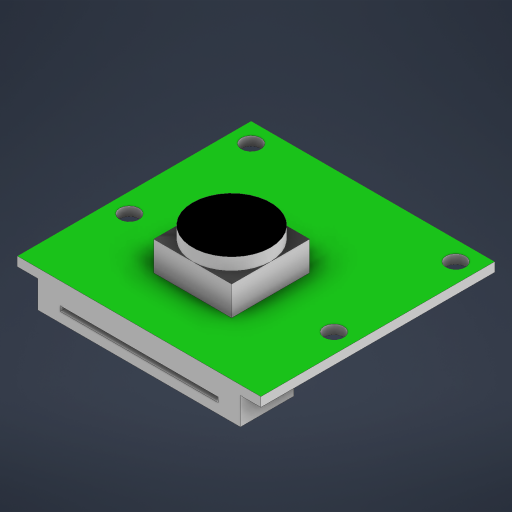
# Autodesk Inventor part: r_camera v2
Saved by Autodesk Inventor 2024.2 (Build 282272000, 272)
## iProperties
Created: 2023-06-18
Part Number: r_camera v2
Material: 일반
Document SubType Name: Modeling
Designer: 6gioc
Density: 1 g/cm^3
Appearance: 기본값
Mass: 1.10891 g
Surface Area: 16.6674 cm^2
Volume: 1.10891 cm^3
Author: 6gioc
Autodesk Inventor part; units mm, degrees
ref_plane "YZ Plane" through (0, 0, 0) normal (1, 0, 0) x (0, 1, 0)
ref_plane "XZ Plane" through (0, 0, 0) normal (0, 1, 0) x (-1, 0, 0)
ref_plane "XY Plane" through (0, 0, 0) normal (0, 0, 1) x (1, 0, 0)
sketch "스케치1" plane through (0, 0, 0) normal (0, 1, 0) x (-1, 0, 0)
  line L0 (0, 0) -> (-25, 0)
  line L1 (-25, 0) -> (-25, -24)
  line L2 (-25, -24) -> (0, -24)
  line L3 (0, -24) -> (0, 0)
  circle A0 centre (-2, -22) radius 1
  circle A1 centre (-23, -22) radius 1
  circle A2 centre (-23, -9.5) radius 1
  circle A3 centre (-2, -9.5) radius 1
  line L4 (-8.5, -13.5) -> (-16.5, -13.5)
  line L5 (-16.5, -13.5) -> (-16.5, -5.5)
  line L6 (-16.5, -5.5) -> (-8.5, -5.5)
  line L7 (-8.5, -5.5) -> (-8.5, -13.5)
  circle A4 centre (-12.5, -9.5) radius 4
  line L8 (-2.1, 0) -> (-22.9, 0)
  line L9 (-22.9, 0) -> (-22.9, -5.5)
  line L10 (-22.9, -5.5) -> (-2.1, -5.5)
  line L11 (-2.1, -5.5) -> (-2.1, 0)
  point P0 (-12.5, 0)
  point P1 (-16.5, -9.5)
  point P2 (-12.5, -5.5)
  point P3 (-8.5, -9.5)
  point P4 (-12.5, -13.5)
  dimension "d0" = 25
  dimension "d1" = 24
  dimension "d2" = 2
  dimension "d3" = 2
  dimension "d4" = 2
  dimension "d5" = 2
  dimension "d6" = 2
  dimension "d8" = 2
  dimension "d9" = 2
  dimension "d10" = 2
  dimension "d12" = 2
  dimension "d15" = 12.5
  dimension "d16" = 9.5
  dimension "d17" = 2
  dimension "d18" = 12.5
  dimension "d19" = 9.5
  dimension "d20" = 8
  dimension "d21" = 8
  dimension "d22" = 8.5
  dimension "d23" = 8.5
  dimension "d24" = 5.5
  dimension "d25" = 21
  dimension "d26" = 8
  dimension "d27" = 20.8
  dimension "d28" = 5.5
  constraints: 24 end point, 6 parallel, 5 centre point, 3 horizontal, 3 perpendicular, 2 midpoint, 2 tangent
  measures "d0" distance of L2.end L1.end
  measures "d1" distance of L1.end L0.end
  measures "d2" diameter of A0
  measures "d3" diameter of A1
  measures "d4" diameter of A2
  measures "d5" diameter of A3
  measures "d6" distance from line of L3 A0.centre
  measures "d8" distance from line of L1 A1.centre
  measures "d9" distance from line of A1.centre L2
  measures "d10" distance from line of L3 A3.centre
  measures "d12" distance from line of L1 A2.centre
  measures "d15" distance of A3.centre A0.centre
  measures "d16" distance from line of L0 A3.centre
  measures "d17" distance from line of L2 A0.centre
  measures "d18" distance of A1.centre A2.centre
  measures "d19" distance from line of L0 A2.centre
  measures "d20" distance of L5.end L6.end
  measures "d21" distance of L4.end L5.end
  measures "d22" distance between parallel lines of L3 L7
  measures "d23" distance between parallel lines of L1 L5
  measures "d24" distance between parallel lines of L0 L6
  measures "d25" distance of A1.centre A0.centre
  measures "d26" diameter of A4
  measures "d27" distance of L10.end L9.end
  measures "d28" distance of L9.end L8.end
extrude "돌출1" add sketch "스케치1" along normal blind 0.95 contours L3 L2 L1 L0 L9 L10 L5 L4 L7 L11 | L11 L10 L6 L9 L0
extrude "돌출2" add sketch "스케치1" along normal blind 3.95 contours L7 A4 L6 | L6 A4 L5 | L7 L4 A4 | A4 L4 L5
extrude "돌출3" add sketch "스케치1" along normal blind 5.2 contours A4
extrude "돌출4" add sketch "스케치1" against normal blind 2.8 contours L11 L10 L6 L9 L0
sketch "스케치2" plane through (0, 0.95, 0) normal (0, 0, 1) x (1, 0, 0)
  line L0 (4.4, -2.22) -> (20.6, -2.22)
  line L1 (20.6, -2.22) -> (20.6, -2.72)
  line L2 (20.6, -2.72) -> (4.4, -2.72)
  line L3 (4.4, -2.72) -> (4.4, -2.22)
  line L4 (0, -0.95) -> (2.1, -0.95) projected
  line L5 (2.1, -0.95) -> (2.1, -3.75) projected
  line L6 (22.9, -0.95) -> (22.9, -3.75) projected
  point P0 (4.4, -2.47)
  point P1 (20.6, -2.47)
  dimension "d37" = 16.2
  dimension "d38" = 0.5
  dimension "d39" = 1.27
  dimension "d40" = 2.3
  dimension "d41" = 2.3
  dimension "d42" = 2.1
  constraints: 8 end point, 2 midpoint, 2 parallel, 1 horizontal, 1 perpendicular
  measures "d37" distance of L1.end L2.end
  measures "d38" distance of L0.end L1.end
  measures "d39" distance between parallel lines of L0 L4
  measures "d40" distance from line of L5 point (4.4, -2.47)
  measures "d41" distance from line of L6 point (20.6, -2.47)
  measures "d42" distance of L4.start L4.end
extrude "돌출5" cut sketch "스케치2" against normal blind 3
